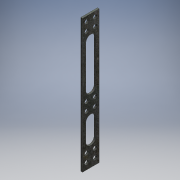
# Autodesk Inventor part: sideLongitudinal
Saved by Autodesk Inventor 2016 (Build 200138000, 138)
## iProperties
Created: 2015-12-25
Part Number: sideLongitudinal
Material: Steel
Document SubType Name: Modeling
Designer: Artur
Density: 7.85 g/cm^3
Appearance: Plate
Mass: 27.6035 g
Surface Area: 49.5216 cm^2
Volume: 3.51637 cm^3
Author: Artur
Autodesk Inventor part; units mm, degrees
ref_plane "YZ Plane" through (0, 0, 0) normal (1, 0, 0) x (0, 1, 0)
ref_plane "XZ Plane" through (0, 0, 0) normal (0, 1, 0) x (-1, 0, 0)
ref_plane "XY Plane" through (0, 0, 0) normal (0, 0, 1) x (1, 0, 0)
sketch "Sketch1" plane through (0, 0, 0) normal (1, 0, 0) x (0, 1, 0)
  line L0 (0, 0) -> (20, 0)
  line L1 (20, 0) -> (20, -160)
  line L2 (20, -160) -> (0, -160)
  line L3 (0, -160) -> (0, 0)
  line L4 (10, 0) -> (10, -160) construction
  line L5 (20, -6) -> (0, -6) construction
  line L6 (20, -16) -> (0, -16) construction
  line L7 (20, -142.5) -> (0, -142.5) construction
  line L8 (25, -152.5) -> (0, -152.5) construction
  line L9 (20, -89) -> (0, -89) construction
  line L10 (25, -99) -> (0, -99) construction
  point P0 (15, -16)
  point P1 (15, -6)
  point P2 (5, -16)
  point P3 (5, -6)
  point P4 (15, -152.5)
  point P5 (15, -142.5)
  point P6 (5, -142.5)
  point P7 (5, -152.5)
  point P8 (15, -99)
  point P9 (15, -89)
  point P10 (5, -89)
  point P11 (5, -99)
  dimension "d1" = 20
  dimension "d10" = 6
  dimension "d11" = 10
  dimension "d12" = 10
  dimension "d13" = 10
  dimension "d14" = 10
  dimension "d16" = 10
  dimension "d17" = 10
  dimension "d27" = 10
  dimension "d28" = 10
  dimension "d29" = 10
  dimension "d30" = 89
  dimension "d40" = 142.5
  dimension "d41" = 160
  constraints: 22 end point, 12 point on line, 6 symmetric about line, 4 horizontal, 2 midpoint, 2 parallel, 2 perpendicular
  measures "d1" distance of L1.end L2.end
  measures "d10" distance between parallel lines of L0 L5
  measures "d11" distance between parallel lines of L5 L6
  measures "d12" diameter of point (15, -16) L4
  measures "d13" diameter of point (15, -6) L4
  measures "d14" distance between parallel lines of L7 L8
  measures "d16" diameter of point (15, -142.5) L4
  measures "d17" diameter of point (15, -152.5) L4
  measures "d27" distance between parallel lines of L9 L10
  measures "d28" diameter of point (15, -99) L4
  measures "d29" diameter of point (15, -89) L4
  measures "d30" distance between parallel lines of L0 L9
  measures "d40" vertical distance of L0.end point (15, -142.5)
  measures "d41" distance of L1.end L0.end
extrude "Extrusion1" add sketch "Sketch1" along normal blind 2
hole "Hole1" at (0, 15, -16) at (0, 15, -6) at (0, 5, -16) at (0, 5, -6) at (0, 15, -142.5) at (0, 15, -152.5) at (0, 5, -152.5) at (0, 5, -142.5) at (0, 15, -89) at (0, 15, -99) at (0, 5, -99) at (0, 5, -89) direction (1, 0, 0) diameter 5 end through all
sketch "Sketch2" plane through (2, 0, 0) normal (1, 0, 0) x (0, 0, -1)
  arc A0 (27.5, 16) -> (27.5, 4) centre (27.5, 10) ccw
  line L0 (27.5, 10) -> (27.5, 4) construction
  line L1 (27.5, 10) -> (27.5, 16) construction
  line L2 (0, 20) -> (0, 0) projected
  line L3 (0, 10) -> (160, 10) construction
  line L4 (160, 0) -> (160, 20) projected
  line L5 (27.5, 16) -> (77.5, 16)
  line L6 (27.5, 4) -> (77.5, 4)
  circle A1 centre (89, 15) radius 2.5 construction
  circle A2 centre (89, 5) radius 2.5 construction
  line L7 (89, 15) -> (89, 5) construction
  circle A3 centre (16, 15) radius 2.5 construction
  circle A4 centre (16, 5) radius 2.5 construction
  line L8 (16, 15) -> (16, 5) construction
  circle A5 centre (99, 15) radius 2.5 construction
  line L9 (99, 15) -> (89, 15) construction
  line L10 (94, 15) -> (94, -7.3428) construction
  arc A6 (77.5, 4) -> (77.5, 16) centre (77.5, 10) ccw
  line L11 (77.5, 10) -> (77.5, 4) construction
  line L12 (77.5, 10) -> (77.5, 16) construction
  line L13 (110.5, 4) -> (131, 4)
  line L14 (131, 16) -> (110.5, 16)
  arc A7 (110.5, 16) -> (110.5, 4) centre (110.5, 10) ccw
  arc A8 (131, 4) -> (131, 16) centre (131, 10) ccw
  circle A9 centre (99, 5) radius 2.5 construction
  circle A10 centre (16, 15) radius 2.5 construction
  circle A11 centre (142.5, 5) radius 2.5 construction
  dimension "d31" = 180
  dimension "d32" = 6
  dimension "d33" = 50
  dimension "d34" = 73
  dimension "d36" = 180
  dimension "d42" = 6
  dimension "d43" = 6
  dimension "d44" = 20.5
  dimension "d46" = 180
  dimension "d47" = 5
  dimension "d48" = 11.5
  dimension "d49" = 43.5
  dimension "d50" = 11.5
  constraints: 26 end point, 8 point on circle, 5 horizontal, 4 centre point, 3 midpoint, 3 vertical, 2 point on line, 2 tangent, 1 parallel, 1 perpendicular
  measures "d31" angle of L0 L1
  measures "d32" distance of L1.end L0.start
  measures "d33" distance of L0.end L6.end
  measures "d34" distance of L7.end L8.end
  measures "d36" angle of L11 L12
  measures "d42" radius of A7
  measures "d43" radius of A8
  measures "d44" distance of L14.start L14.end
  measures "d47" diameter of A3
  measures "d48" horizontal distance of L0.start L8.start
  measures "d49" distance of A9.centre A11.centre
  measures "d50" horizontal distance of A9.centre A7.centre
extrude "Extrusion2" cut sketch "Sketch2" against normal blind 10
equation "\"d13\" = d12"
equation "\"d16\" = d12"
equation "\"d17\" = d12"
equation "\"d28\" = d27"
equation "\"d29\" = d12"
equation "\"d42\" = d32"
equation "\"d43\" = d32"
equation "\"d46\" = d36"
equation "\"d48\" = 0 * d47 + 0.5 * d34 - 0.5 * d33"
equation "\"d50\" = -0.5 * d44 + 0.5 * d49 + 0 * d47"
body "Solid1"
